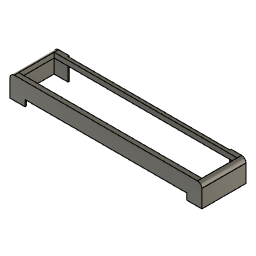
jarvis-controller-cover v4 (Autodesk Fusion 360 design; units mm, degrees)
Autodesk Fusion 360 part; units mm, degrees
sketch "top" plane through (0, 0, 0) normal (0, 0, 1) x (1, 0, 0)
  line L0 (0, 0) -> (150, 0)
  line L1 (150, 0) -> (150, 33)
  line L2 (150, 33) -> (0, 33)
  line L3 (0, 33) -> (0, 0)
  line L4 (-1, -1) -> (151, -1)
  line L5 (151, -1) -> (151, 34)
  line L6 (151, 34) -> (-1, 34)
  line L7 (-1, 34) -> (-1, -1)
  line L8 (2.5, 2.5) -> (147.5, 2.5)
  line L9 (147.5, 2.5) -> (147.5, 30.5)
  line L10 (147.5, 30.5) -> (2.5, 30.5)
  line L11 (2.5, 30.5) -> (2.5, 2.5)
  line L12 (11, 30.5) -> (11, 34)
  line L13 (-1, 16.5) -> (151, 16.5) construction
  line L14 (75, 34) -> (75, -1) construction
  line L15 (139, 30.5) -> (139, 34)
  line L16 (11, 2.5) -> (11, -1)
  line L17 (139, 2.5) -> (139, -1)
  dimension "d4" = 150
  dimension "d5" = 33
  dimension "d6" = 1
  dimension "d7" = -2.5
  dimension "d8" = 12
  constraint horizontal L0
  constraint vertical L1
  constraint horizontal L2
  constraint vertical L3
  constraint coincident L0.start L3.end
  constraint coincident L10 L12.start
  constraint coincident L6 L12.end
  constraint perpendicular L6 L12
  constraint midpoint L7 L13.start
  constraint midpoint L5 L13.end
  constraint midpoint L6 L14.start
  constraint midpoint L4 L14.end
  constraint symmetric L12.start L14 L15.start
  constraint symmetric L12.end L14 L15.end
  constraint symmetric L12.start L13 L16.start
  constraint symmetric L12.end L13 L16.end
  constraint symmetric L13 L15.start L17.start
  constraint symmetric L13 L15.end L17.end
  measures "d4" distance of L0.start L0.end
  measures "d5" distance of L0.start L2.end
  measures "d8" distance of L7 L12
extrude "Extrude1" add sketch "top" against normal blind 15 contours L0 L2 L3 L4 L6 L7 L12 L16 | L0 L1 L2 L4 L5 L6 L15 L17 makes body 1 at (-1, 22.3333, -5) makes body 2 at (151, 10.6667, -5)
extrude "Extrude2" add sketch "top" against normal blind 10 contours L0 L4 L16 L17 bodies 1 2
extrude "Extrude3" add sketch "top" against normal blind 1.5 contours L0 L2 L3 L8 L10 L11 L12 L16 | L0 L8 L16 L17 | L0 L1 L2 L8 L9 L10 L15 L17 | L2 L10 L12 L15 bodies 1
extrude "Extrude4" add sketch "top" along normal blind 2.5 contours L0 L2 L3 L8 L10 L11 L12 L16 | L0 L2 L3 L4 L6 L7 L12 L16 | L0 L8 L16 L17 | L0 L4 L16 L17 | L0 L1 L2 L8 L9 L10 L15 L17 | L0 L1 L2 L4 L5 L6 L15 L17 | L2 L10 L12 L15 bodies 1
fillet "Fillet1" radius 3.5 2 edges at (151, 16.5, 2.5) (-1, 16.5, 2.5) on bodies 1
named bodies: "cover"
